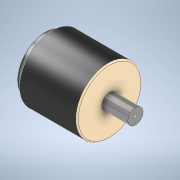
# Autodesk Inventor part: Motor
Saved by Autodesk Inventor 2021 (Build 250183000, 183)
## iProperties
Created: 2021-02-20
Part Number: Motor
Material: Generic
Document SubType Name: Modeling
Designer: Krishmulls
Density: 1 g/cm^3
Appearance: Default
Author: Krishmulls
Autodesk Inventor part; units mm, degrees
ref_plane "YZ Plane" through (0, 0, 0) normal (1, 0, 0) x (0, 1, 0)
ref_plane "XZ Plane" through (0, 0, 0) normal (0, 1, 0) x (-1, 0, 0)
ref_plane "XY Plane" through (0, 0, 0) normal (0, 0, 1) x (1, 0, 0)
sketch "Sketch3" plane through (0, 0, 0) normal (1, 0, 0) x (0, 1, 0)
  circle A0 centre (0, 0) radius 11.7
  dimension "d1" = 23.4
  constraints: 1 centre point, 1 coincident
  measures "d1" diameter of A0
extrude "Extrusion1" add sketch "Sketch3" along normal mid plane 90
sketch "Sketch4" plane through (45, 0, 0) normal (1, 0, 0) x (0, 0, -1)
  point P0 (0, 0)
sketch "Sketch5" plane through (-45, 0, 0) normal (-1, 0, 0) x (0, 0, 1)
  circle A0 centre (0, 0) radius 11.7 projected
  circle A1 centre (0, 0) radius 50
  dimension "d4" = 100
  constraints: 1 centre point, 1 coincident
  measures "d4" diameter of A1
extrude "Extrusion2" add sketch "Sketch5" along normal mid plane 100 contours A0 | A1
sketch "Sketch6" plane through (-95, 0, 0) normal (-1, 0, 0) x (0, 0, 1)
  circle A0 centre (0, 0) radius 11.7 projected
  circle A1 centre (0, 0) radius 43.0072
  circle A2 centre (0, 0) radius 50
  constraints: 2 centre point, 2 coincident
extrude "Extrusion3" cut sketch "Sketch6" against normal blind 10 contours A2
fillet "Fillet1" radius 2 1 edges at (-85, 0, -50)
fillet "Fillet2" radius 2 1 edges at (-95, 0, -43.0072)
thread "Thread1" size "M90x6" class "6g" standard "ANSI Metric M Profile" full length
fillet "Fillet3" radius 2 1 edges at (5, 0, -50)
body "Solid1"
